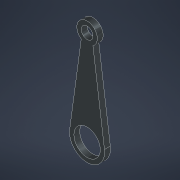
# Autodesk Inventor part: P012-Bielle
Saved by Autodesk Inventor 2021.3 (Build 253353000, 353)
## iProperties
Company: HES-SO
Created: 2022-03-31
Part Number: P012-Bielle
Material: Iron, Gray
Document SubType Name: Modeling
Designer: Rémi & Elise
Density: 7.15 g/cm^3
Appearance: Iron Gray
Mass: 42.1506 g
Surface Area: 38.2752 cm^2
Volume: 5.8952 cm^3
Author: Rémi & Elise
Title: Bielle
Autodesk Inventor part; units mm, degrees
ref_plane "YZ Plane" through (0, 0, 0) normal (1, 0, 0) x (0, 1, 0)
ref_plane "XZ Plane" through (0, 0, 0) normal (0, 1, 0) x (-1, 0, 0)
ref_plane "XY Plane" through (0, 0, 0) normal (0, 0, 1) x (1, 0, 0)
sketch "Sketch2" plane through (0, 0, 0) normal (0, 1, 0) x (-1, 0, 0)
  line L0 (0, -28.76) -> (0, 88.56) construction
  circle A0 centre (0, 64.8) radius 4
  arc A1 (4, 59.0554) -> (-4, 59.0554) centre (0, 64.8) ccw
  line L1 (-4, 59.0554) -> (-11.8883, 1.6332)
  line L2 (11.8883, 1.6332) -> (4, 59.0554)
  circle A2 centre (0, 0) radius 9
  arc A3 (-11.8883, 1.6332) -> (11.8883, 1.6332) centre (0, 0) ccw
  dimension "d7" = 3
  dimension "d8" = 8
  dimension "d22" = 64.8
  dimension "d25" = 3
  dimension "d26" = 18
  dimension "d27" = 8
  constraints: 4 centre point, 4 end point, 4 point on circle, 3 coincident, 2 horizontal alignment, 1 point on line, 1 tangent
  measures "d7" radial gap between concentric circles of A0 A1
  measures "d8" diameter of A0
  measures "d22" distance of point (0, 0) A0.centre
  measures "d25" radial gap between concentric circles of A3 A2
  measures "d26" diameter of A2
  measures "d27" distance of L1.start L2.end
extrude "Extrusion1" add sketch "Sketch2" along normal blind 4
body "Solid1"
